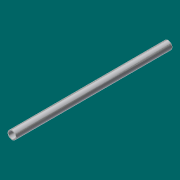
# Autodesk Inventor part: A1-18002-100-22 2.25in x 5ft bar tube
Saved by Autodesk Inventor 2017 (Build 210142000, 142)
## iProperties
Created: 2018-01-23
Part Number: A1-18002-100-22 2.25in x 5ft bar tube
Material: PVC-Piping
Document SubType Name: Modeling
Designer: Graeme_Van_Dongen
Density: 1.4 g/cm^3
Appearance: Smooth - White
Mass: 2120.86 g
Surface Area: 5898.01 cm^2
Volume: 1514.9 cm^3
Description: 2 1/2" STD x 54 1/4" PIPE, PVC
Author: Graeme_Van_Dongen
Autodesk Inventor part; units mm, degrees
ref_plane "YZ Plane" through (0, 0, 0) normal (1, 0, 0) x (0, 1, 0)
ref_plane "XZ Plane" through (0, 0, 0) normal (0, 1, 0) x (-1, 0, 0)
ref_plane "XY Plane" through (0, 0, 0) normal (0, 0, 1) x (1, 0, 0)
sketch "Sketch1" plane through (0, 0, 0) normal (0, 0, 1) x (1, 0, 0)
  circle A0 centre (0, 0) radius 36.5125
  circle A1 centre (0, 0) radius 31.3563
  dimension "d0" = 73.025
  dimension "d1" = 62.7126
  constraints: 2 centre point, 2 coincident
  measures "d0" diameter of A0
  measures "d1" diameter of A1
extrude "Extrusion1" add sketch "Sketch1" along normal blind 1377.95
body "Solid1"
